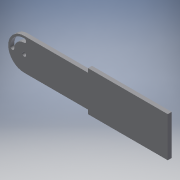
# Autodesk Inventor part: Posicionador
Saved by Autodesk Inventor 2018 (Build 220112000, 112)
## iProperties
Created: 2021-07-05
Part Number: Posicionador
Material: Genérico
Document SubType Name: Modeling
Designer: GABRIEL
Density: 1 g/cm^3
Appearance: Valor por defecto
Author: GABRIEL
Autodesk Inventor part; units mm, degrees
ref_plane "YZ Plane" through (0, 0, 0) normal (1, 0, 0) x (0, 1, 0)
ref_plane "XZ Plane" through (0, 0, 0) normal (0, 1, 0) x (-1, 0, 0)
ref_plane "XY Plane" through (0, 0, 0) normal (0, 0, 1) x (1, 0, 0)
sketch "Boceto1" plane through (0, 0, 0) normal (0, 1, 0) x (-1, 0, 0)
  line L0 (-320, 0) -> (-320, -140)
  circle A0 centre (-50, -70) radius 5
  circle A1 centre (-50, -30) radius 5
  circle A2 centre (-10, -70) radius 5
  arc A3 (-15, -70) -> (-50, -35) centre (-50, -70) ccw
  arc A4 (-5, -70) -> (-50, -25) centre (-50, -70) ccw
  line L1 (-140, -140) -> (-140, 0)
  circle A5 centre (-50, -70) radius 50
  line L2 (-140, -20) -> (-50, -20)
  line L3 (-140, -120) -> (-50, -120)
  line L4 (-140, -140) -> (-320, -140)
  line L5 (-320, 0) -> (-140, 0)
  point P0 (0, 0)
  dimension "d1" = 140
  dimension "d10" = 10
  dimension "d11" = 10
  dimension "d14" = 10
  dimension "d22" = 40
  dimension "d23" = 40
  dimension "d25" = 35
  dimension "d26" = 45
  dimension "d29" = 180
  dimension "d43" = 100
  dimension "d45" = 50
  dimension "d50" = 20
  dimension "d51" = 20
  dimension "d52" = 140
  dimension "d53" = 50
  dimension "d54" = 135
  dimension "d55" = 5
  constraints: 12 end point, 10 point on circle, 6 centre point, 5 tangent, 2 horizontal, 2 parallel, 2 point on line, 1 coincident, 1 vertical
  measures "d1" distance of L0.end L0.start
  measures "d10" diameter of A0
  measures "d11" diameter of A1
  measures "d14" diameter of A2
  measures "d22" distance of A2.centre A0.centre
  measures "d23" distance of A1.centre A0.centre
  measures "d25" radius of A3
  measures "d26" radius of A4
  measures "d29" distance between parallel lines of L0 L1
  measures "d43" diameter of A5
  measures "d45" distance from line of L2 A4.centre
  measures "d50" distance between parallel lines of L5 L2
  measures "d51" distance from line of point (0, 0) L2
  measures "d52" distance from line of point (0, 0) L1
  measures "d53" distance from line of A2.end L2
  measures "d54" distance from line of A2.end L1
  measures "d55" distance from line of A1.end L2
extrude "Extrusión2" add sketch "Boceto1" along normal blind 10
